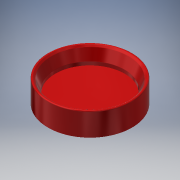
# Autodesk Inventor part: bat
Saved by Autodesk Inventor 2019.3 (Build 233278000, 278)
## iProperties
Created: 2020-09-01
Part Number: bat
Material: ABS-Kunststoff
Document SubType Name: Modeling
Designer: Nicolas Frick
Density: 1.06 g/cm^3
Appearance: Glatt - Weiß
Author: Nicolas Frick
Autodesk Inventor part; units mm, degrees
ref_plane "YZ Plane" through (0, 0, 0) normal (1, 0, 0) x (0, 1, 0)
ref_plane "XZ Plane" through (0, 0, 0) normal (0, 1, 0) x (-1, 0, 0)
ref_plane "XY Plane" through (0, 0, 0) normal (0, 0, 1) x (1, 0, 0)
sketch "Skizze1" plane through (0, 0, 0) normal (0, 1, 0) x (-1, 0, 0)
  circle A0 centre (0, 0) radius 37
  dimension "d0" = 74
  constraints: 1 centre point, 1 coincident
  measures "d0" diameter of A0
extrude "Extrusion1" add sketch "Skizze1" along normal blind 20.5
sketch "Skizze2" plane through (0, 20.5, 0) normal (0, 1, 0) x (1, 0, 0)
  circle A0 centre (0, 0) radius 30.5
  dimension "d3" = 61
  constraints: 1 centre point, 1 coincident
  measures "d3" diameter of A0
extrude "Extrusion2" cut sketch "Skizze2" against normal blind 13
chamfer "Fase1" distance 5 angle 45 1 edges at (-30.5, 20.5, 0)
chamfer "Fase2" distance 5 angle 45 1 edges at (-30.5, 15.5, 0)
fillet "Rundung2" radius 1 2 edges at (37, 20.5, 0) (-35.5, 20.5, 0)
fillet "Rundung3" radius 1 2 edges at (-34.0355, 19.0355, 0) (-30.5, 10.5, 0)
